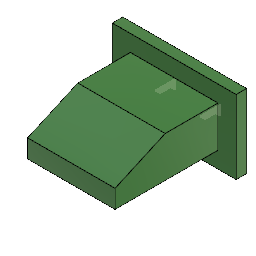
Connecteur_Thermocouple_femelle (Autodesk Fusion 360 design; units mm, degrees)
Autodesk Fusion 360 part; units mm, degrees
sketch "Esquisse1" plane through (0, 0, 0) normal (1, 0, 0) x (0, 1, 0)
  line L0 (0, 0) -> (19.5, 0)
  line L1 (19.5, 0) -> (19.5, 7.75)
  line L2 (19.5, 7.75) -> (9.5, 7.75)
  line L3 (9.5, 7.75) -> (0, 3.5)
  line L4 (0, 3.5) -> (0, 0)
  dimension "d1" = 7.75
  dimension "d2" = 19.5
  dimension "d3" = 10
  dimension "d4" = 3.5
  constraint coincident L0.start L4.end
  constraint horizontal L0
  constraint perpendicular L0 L1
  constraint perpendicular L1 L2
  constraint perpendicular L0 L4
  measures "d1" distance of L0.end L1.end
  measures "d2" distance of L0.start L0.end
  measures "d3" distance of L1.end L2.end
  measures "d4" distance of L3.end L0.start
extrude "Extrusion1" add sketch "Esquisse1" along normal blind 16.6
sketch "Esquisse2" plane through (0, 19.5, 0) normal (0, 1, 0) x (-1, 0, 0)
  line L0 (0, 0) -> (0, 7.75)
  line L1 (0, 7.75) -> (-16.6, 7.75)
  line L2 (-16.6, 7.75) -> (-16.6, 0)
  line L3 (-16.6, 0) -> (0, 0)
  line L4 (-20.05, 10.875) -> (3.45, 10.875)
  line L5 (3.45, 10.875) -> (3.45, -3.125)
  line L6 (3.45, -3.125) -> (-20.05, -3.125)
  line L7 (-20.05, -3.125) -> (-20.05, 10.875)
  dimension "d7" = 23.5
  dimension "d8" = 14
  dimension "d9" = 3.45
  dimension "d10" = 3.125
  constraint horizontal L4
  constraint vertical L5
  constraint horizontal L6
  constraint vertical L7
  measures "d7" distance of L5.end L6.end
  measures "d8" distance of L4.end L5.end
  measures "d9" distance of L0 L5
  measures "d10" distance of L1 L4
extrude "Extrusion2" add sketch "Esquisse2" along normal blind 2 contours L0 L1 L2 L3 | L4 L5 L6 L7
sketch "Esquisse3" plane through (0, 21.5, 0) normal (0, 1, 0) x (-1, 0, 0)
  line L0 (-20.05, -3.125) -> (3.45, -3.125)
  line L1 (3.45, -3.125) -> (3.45, 10.875)
  line L2 (3.45, 10.875) -> (-20.05, 10.875)
  line L3 (-20.05, 10.875) -> (-20.05, -3.125)
  line L4 (-8.3, 10.875) -> (-8.3, -3.125)
  line L5 (-14.05, 0.875) -> (-11.05, 0.875)
  line L6 (-11.05, 0.875) -> (-11.05, 3.875)
  line L7 (-11.05, 3.875) -> (-10.05, 3.875)
  line L8 (-10.05, 3.875) -> (-10.05, 5.875)
  line L9 (-10.05, 5.875) -> (-15.05, 5.875)
  line L10 (-15.05, 5.875) -> (-15.05, 3.875)
  line L11 (-15.05, 3.875) -> (-14.05, 3.875)
  line L12 (-14.05, 3.875) -> (-14.05, 0.875)
  line L13 (-1.55, 3.875) -> (-2.55, 3.875)
  line L14 (-6.55, 5.875) -> (-1.55, 5.875)
  line L15 (-6.55, 3.875) -> (-6.55, 5.875)
  line L16 (-5.55, 3.875) -> (-6.55, 3.875)
  line L17 (-5.55, 0.875) -> (-5.55, 3.875)
  line L18 (-2.55, 0.875) -> (-5.55, 0.875)
  line L19 (-2.55, 3.875) -> (-2.55, 0.875)
  line L20 (-1.55, 5.875) -> (-1.55, 3.875)
  line L21 (-14.05, 3.875) -> (-11.05, 3.875)
  line L22 (-2.55, 3.875) -> (-5.55, 3.875)
  dimension "d14" = 5
  dimension "d15" = 2
  dimension "d16" = 5
  dimension "d17" = 3
  dimension "d18" = 5
  dimension "d19" = 5
  constraint midpoint L2 L4.start
  constraint midpoint L0 L4.end
  constraint perpendicular L4 L5
  constraint perpendicular L5 L6
  constraint perpendicular L6 L7
  constraint perpendicular L5 L8
  constraint perpendicular L8 L9
  constraint perpendicular L9 L10
  constraint perpendicular L10 L11
  constraint perpendicular L5 L12
  constraint equal L7 L11
  constraint equal L8 L10
  constraint symmetric L4 L5.start L18.start
  constraint symmetric L4 L5.end L17.start
  constraint symmetric L4 L6.end L16.start
  constraint symmetric L4 L7.end L15.start
  constraint symmetric L4 L8.end L14.start
  constraint symmetric L4 L9.end L14.end
  constraint symmetric L4 L10.end L13.start
  constraint symmetric L4 L11.end L13.end
  measures "d14" distance of L8.end L9.end
  measures "d15" distance of L9.end L10.end
  measures "d16" distance of L5 L9
  measures "d17" distance of L5.start L5.end
  measures "d18" distance of L3 L10
  measures "d19" distance of L2 L9
extrude "Extrusion3" cut sketch "Esquisse3" against normal blind 2 contours L5 L6 L12 L21 | L7 L8 L9 L10 L11 L21 | L13 L14 L15 L16 L20 L22 | L17 L18 L19 L22
sketch "Esquisse4" plane through (0, 21.5, 0) normal (0, 1, 0) x (-1, 0, 0)
  line L0 (-11.05, 0.875) -> (-14.05, 0.875)
  line L1 (-14.05, 0.875) -> (-14.05, 3.875)
  line L2 (-14.05, 3.875) -> (-15.05, 3.875)
  line L3 (-15.05, 3.875) -> (-15.05, 5.875)
  line L4 (-15.05, 5.875) -> (-10.05, 5.875)
  line L5 (-10.05, 5.875) -> (-10.05, 3.875)
  line L6 (-10.05, 3.875) -> (-11.05, 3.875)
  line L7 (-11.05, 3.875) -> (-11.05, 0.875)
  line L8 (-6.55, 3.875) -> (-6.55, 5.875)
  line L9 (-6.55, 5.875) -> (-1.55, 5.875)
  line L10 (-1.55, 5.875) -> (-1.55, 3.875)
  line L11 (-1.55, 3.875) -> (-2.55, 3.875)
  line L12 (-2.55, 3.875) -> (-2.55, 0.875)
  line L13 (-2.55, 0.875) -> (-5.55, 0.875)
  line L14 (-5.55, 0.875) -> (-5.55, 3.875)
  line L15 (-5.55, 3.875) -> (-6.55, 3.875)
  line L16 (-20.05, -3.125) -> (3.45, -3.125)
  line L17 (3.45, -3.125) -> (3.45, 10.875)
  line L18 (3.45, 10.875) -> (-20.05, 10.875)
  line L19 (-20.05, 10.875) -> (-20.05, -3.125)
  line L20 (-15.05, 5.875) -> (-10.05, 5.875)
  line L21 (-10.05, 5.875) -> (-10.05, 3.875)
  line L22 (-10.05, 3.875) -> (-15.05, 3.875)
  line L23 (-15.05, 3.875) -> (-15.05, 5.875)
  line L24 (-6.55, 5.875) -> (-1.55, 5.875)
  line L25 (-1.55, 5.875) -> (-1.55, 3.875)
  line L26 (-1.55, 3.875) -> (-6.55, 3.875)
  line L27 (-6.55, 3.875) -> (-6.55, 5.875)
  constraint horizontal L20
  constraint vertical L21
  constraint horizontal L22
  constraint vertical L23
  constraint coincident L5.end L6.start
  constraint coincident L3.end L4.start
  constraint horizontal L24
  constraint vertical L25
  constraint horizontal L26
  constraint vertical L27
  constraint coincident L10.end L11.start
  constraint coincident L8.end L9.start
extrude "Extrusion4" cut sketch "Esquisse4" against normal blind 5 contours L2 L3 L4 L5 L6 L20 L21 L22 L23 | L8 L9 L10 L11 L15 L24 L25 L26 L27
chamfer "Chanfrein1" [suppressed]
fillet "Congé1" [suppressed]
